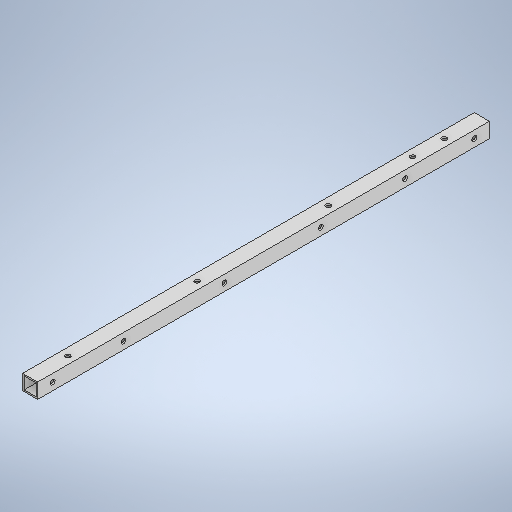
# Autodesk Inventor part: small_kaku_1010_200
Saved by Autodesk Inventor 2025.1 (Build 291241000, 241)
## iProperties
Created: 2024-10-08
Part Number: small_kaku_1010_200
Material: 一般
Document SubType Name: Modeling
Designer: yuki0520
Density: 1 g/cm^3
Appearance: 既定
Author: yuki0520
Autodesk Inventor part; units mm, degrees
ref_plane "YZ Plane" through (0, 0, 0) normal (1, 0, 0) x (0, 1, 0)
ref_plane "XZ Plane" through (0, 0, 0) normal (0, 1, 0) x (-1, 0, 0)
ref_plane "XY Plane" through (0, 0, 0) normal (0, 0, 1) x (1, 0, 0)
sketch "スケッチ1" plane through (0, 0, 0) normal (0, 0, 1) x (1, 0, 0)
  line L0 (5, -5) -> (-5, -5)
  line L1 (-5, -5) -> (-5, 5)
  line L2 (-5, 5) -> (5, 5)
  line L3 (5, 5) -> (5, -5)
  line L4 (5, -5) -> (-5, 5) construction
  line L5 (-5, -5) -> (5, 5) construction
  line L6 (4, 4) -> (-4, 4)
  line L7 (-4, 4) -> (-4, -4)
  line L8 (-4, -4) -> (4, -4)
  line L9 (4, -4) -> (4, 4)
  point P0 (0, 0)
  dimension "d0" = 10
  dimension "d1" = 10
  dimension "d2" = 1
  constraints: 20 end point, 4 parallel, 2 midpoint, 2 perpendicular, 1 horizontal, 3 other
  measures "d0" distance of L1.end L2.end
  measures "d1" distance of L0.end L1.end
  measures "d2" distance between parallel lines of L2 L6
extrude "押し出し1" add sketch "スケッチ1" along normal blind 300
sketch "スケッチ2" plane through (5, -5, 0) normal (1, 0, 0) x (0, 0, -1)
  line L0 (0, 0) -> (0, 10) projected
  line L1 (0, 10) -> (-300, 10) projected
  line L2 (-300, 0) -> (-300, 10) projected
  line L3 (0, 0) -> (-300, 0) projected
  line L4 (0, 5) -> (-300, 5)
  line L5 (-300, 0) -> (-300, 10) projected
  point P0 (-290, 5)
  point P1 (-176, 5)
  point P2 (-56, 5)
  point P3 (-10, 5)
  point P4 (-112, 5)
  point P5 (-243, 5)
  point P6 (-149.5, 5)
  dimension "d7" = 120
  dimension "d25" = 10
  dimension "d26" = 46
  dimension "d27" = 10
  dimension "d28" = 114
  dimension "d29" = 56
  dimension "d34" = 26.5
  dimension "d35" = 93.5
  dimension "d36" = 93.5
  constraints: 2 midpoint, 10 other
  measures "d7" distance of point (-176, 5) point (-56, 5)
  measures "d25" distance from line of L0 point (-10, 5)
  measures "d26" distance of point (-10, 5) point (-56, 5)
  measures "d27" distance of point (-300, 5) point (-290, 5)
  measures "d28" distance of point (-176, 5) point (-290, 5)
  measures "d29" distance of point (-56, 5) point (-112, 5)
  measures "d34" distance of point (-176, 5) point (-149.5, 5)
  measures "d35" distance of point (-149.5, 5) point (-243, 5)
  measures "d36" distance of point (-56, 5) point (-149.5, 5)
hole "穴1" at (5, 0, 290) at (5, 0, 176) at (5, 0, 56) at (5, 0, 10) at (5, 0, 112) at (5, 0, 243) direction (-1, 0, 0) diameter 3.3 end through all
sketch "スケッチ3" plane through (-5, 5, 0) normal (0, 1, 0) x (1, 0, 0)
  line L0 (10, 0) -> (0, 0) projected
  line L1 (0, 0) -> (0, -300) projected
  line L2 (10, -300) -> (0, -300) projected
  line L3 (10, 0) -> (10, -300) projected
  line L4 (5, -300) -> (5, 0)
  point P0 (5, -275)
  point P1 (5, -46)
  point P2 (5, -102)
  point P3 (5, -189)
  point P4 (5, -25)
  dimension "d17" = 25
  dimension "d30" = 46
  dimension "d31" = 56
  dimension "d32" = 87
  dimension "d33" = 25
  constraints: 5 point on line, 2 end point, 1 midpoint, 1 perpendicular
  measures "d17" distance from line of L2 point (5, -275)
  measures "d30" distance from line of L0 point (5, -46)
  measures "d31" distance of point (5, -102) point (5, -46)
  measures "d32" distance of point (5, -102) point (5, -189)
  measures "d33" distance from line of L0 point (5, -25)
hole "穴2" at (0, 5, 275) at (0, 5, 46) at (0, 5, 102) at (0, 5, 189) at (0, 5, 25) direction (0, -1, 0) diameter 3.3 end through all
equation "\"d35\" = d36"
